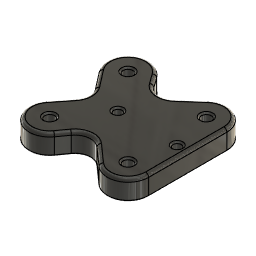
Rod_Clamp_Fixture (Autodesk Fusion 360 design; units mm, degrees)
Autodesk Fusion 360 part; units mm, degrees
note: some values were not read from the file. Set by a fixed rule: which sketch regions a step uses.
sketch "Sketch1" plane through (0, 0, 0) normal (0, 0, 1) x (1, 0, 0)
  circle A0 centre (0, 0) radius 3.125
  circle A1 centre (0, 50) radius 3.125
  circle A2 centre (0, 0) radius 13.125
  circle A3 centre (0, 50) radius 13.125
  line L0 (0, 50) -> (0, 0) construction
  line L1 (37.5, 50.1021) -> (37.5, 0.1021) construction
  line L2 (0, 25) -> (18.55, 25) construction
  circle A4 centre (18.55, 25) radius 2.6
  circle A5 centre (18.55, 25) radius 12.6 construction
  line L3 (-10.2863, 8.1521) -> (-1.9703, 18.6453)
  line L4 (-1.8904, 30.9655) -> (-10.3911, 41.9818)
  arc A6 (-1.9703, 18.6453) -> (-1.8904, 30.9655) centre (-9.8074, 24.8564) ccw
  line L5 (75, 25) -> (56.45, 25) construction
  circle A7 centre (56.45, 25) radius 2.6
  circle A8 centre (56.45, 25) radius 12.6 construction
  line L6 (10.6707, 57.6421) -> (15.1766, 51.3504)
  line L7 (50, 25) -> (50, 37.5) construction
  line L8 (0, 0) -> (37.5, 0) construction
  line L9 (18.55, 25) -> (56.45, 25) construction
  line L10 (37.5, 25) -> (37.5, 37.5) construction
  circle A9 centre (50.0503, 50) radius 13.125
  circle A10 centre (50.0503, 50) radius 3.125
  circle A11 centre (50.0503, 0) radius 13.125
  circle A12 centre (50.0503, 0) radius 3.125
  line L11 (29.9485, 49.6973) -> (41.3329, 59.8118)
  line L12 (21.6444, 42.3194) -> (21.6444, 45)
  line L13 (0, 50) -> (50.0503, 50) construction
  arc A13 (15.1766, 51.3504) -> (29.9485, 49.6973) centre (23.3067, 57.173) ccw
  line L14 (63.1753, 50) -> (63.1753, 0)
  line L15 (56.45, 25) -> (61.45, 25) construction
  arc A14 (29.9485, 0.3027) -> (15.1766, -1.3504) centre (23.3067, -7.173) ccw
  line L16 (10.6707, -7.6421) -> (15.1766, -1.3504)
  line L17 (29.9485, 0.3027) -> (41.3329, -9.8118)
  point P0 (5.95, 25)
  dimension "d156" = 6.25
  dimension "d159" = 25
  dimension "d160" = 25
  dimension "d161" = 10
  dimension "d162" = 10
  dimension "d163" = 50
  dimension "d165" = 50
  dimension "d166" = 18.55
  dimension "d167" = 5.2
  dimension "d168" = 10
  dimension "d169" = 10
  dimension "d178" = 37.5
  dimension "d5" = 25
  dimension "d6" = 25
  dimension "d7" = 10
  dimension "d8" = 10
  dimension "d9" = 6.25
  dimension "d10" = 50
  dimension "d11" = 10
  dimension "d12" = 5
  constraint coincident A0.centre A2.centre
  constraint coincident A1.centre A3.centre
  constraint midpoint L0 L2.start
  constraint vertical L1
  constraint perpendicular L0 L2
  constraint coincident L2.end A4.centre
  constraint coincident A2 L3.start
  constraint tangent A2 L3
  constraint coincident A5 P0
  constraint coincident A3 L4.end
  constraint tangent A3 L4
  constraint tangent L4 A6
  constraint tangent L3 A6
  constraint symmetric L1 L2.end L5.end
  constraint symmetric L1 A4 A7
  constraint symmetric L1 A5 A8
  constraint tangent A5 L6
  constraint coincident A3 L6.start
  constraint tangent A3 L6
  constraint perpendicular L1 L8
  constraint coincident L1 L8.end
  constraint midpoint L9 L10.start
  constraint coincident A9 L11.end
  constraint tangent A9 L11
  constraint vertical L12
  constraint coincident A9.centre A10.centre
  constraint perpendicular L0 L13
  constraint coincident L6 L12.start
  constraint coincident L12.start L11
  constraint tangent L6 A13
  constraint tangent L11 A13
  constraint coincident A9 L14.start
  constraint coincident A11 L14.end
  constraint tangent A11 L14
  constraint coincident L5.end A7.centre
  constraint perpendicular L14 L15
  constraint symmetric L2 L6.start L16.start
  constraint symmetric L2 L11.end L17.end
  constraint symmetric L2 L6.end A14.end
  constraint symmetric L2 L11.start A14.start
  constraint symmetric L2 A13 A14
  constraint tangent A9 L14
  measures "d156" diameter of A0
  measures "d163" distance of A1.centre A0.centre
  measures "d165" distance of L2.start L7.start
  measures "d166" distance of L2.start L2.end
  measures "d167" diameter of A4
  measures "d169" radius of A6
  measures "d178" distance of A0.centre L8.end
  measures "d9" diameter of A12
  measures "d10" distance of A9.centre A11.centre
  measures "d11" radius of A13
  measures "d12" distance of L5.end L15.end
extrude "Extrude1" add sketch "Sketch1" along normal blind 12.5
chamfer "Chamfer1" distance 1 angle 45 6 edges at (-2.9135, 51.13, 12.5) (47.1368, 51.13, 12.5) (54.0259, 25.9402, 12.5) (16.1259, 25.9402, 12.5) (47.1368, 1.13, 12.5) (-2.9135, 1.13, 12.5)
fillet "Fillet1" radius 2 14 edges at (12.9237, 54.4962, 12.5) (-7.8314, 60.5326, 12.5) (-6.1408, 36.4737, 12.5) (0.1923, 24.7916, 12.5) (-6.1283, 13.3987, 12.5) (-7.8994, -10.4816, 12.5) (12.9237, -4.4962, 12.5) (22.1945, 2.765, 12.5) (35.6407, -4.7546, 12.5) (55.4285, -11.9725, 12.5) (63.1753, 25, 12.5) (22.1945, 47.235, 12.5) (35.6407, 54.7546, 12.5) (55.4285, 61.9725, 12.5)
sketch "Sketch2" plane through (0, 0, 0) normal (0, 0, -1) x (1, 0, 0)
  circle A0 centre (0, 0) radius 3.125
  line L0 (22.6, -22.6617) -> (18.55, -20.3235)
  line L1 (18.55, -20.3235) -> (14.5, -22.6617)
  line L2 (14.5, -22.6617) -> (14.5, -27.3383)
  line L3 (14.5, -27.3383) -> (18.55, -29.6765)
  line L4 (18.55, -29.6765) -> (22.6, -27.3383)
  line L5 (22.6, -27.3383) -> (22.6, -22.6617)
  circle A1 centre (50.0503, 0) radius 3.125
  circle A2 centre (0, -50) radius 3.125
  circle A3 centre (56.45, -25) radius 2.6
  circle A4 centre (50.0503, -50) radius 3.125
  circle A5 centre (18.55, -25) radius 2.6
  arc A6 (10.6707, 7.6421) -> (-10.2863, -8.1521) centre (0, 0) ccw
  line L6 (-10.2863, -8.1521) -> (-1.9703, -18.6453)
  arc A7 (-1.8904, -30.9655) -> (-1.9703, -18.6453) centre (-9.8074, -24.8564) ccw
  line L7 (-1.8904, -30.9655) -> (-10.3911, -41.9818)
  arc A8 (-10.3911, -41.9818) -> (10.6707, -57.6421) centre (0, -50) ccw
  line L8 (10.6707, -57.6421) -> (15.1766, -51.3504)
  arc A9 (29.9485, -49.6973) -> (15.1766, -51.3504) centre (23.3067, -57.173) ccw
  line L9 (29.9485, -49.6973) -> (41.3329, -59.8118)
  arc A10 (41.3329, -59.8118) -> (63.1753, -50) centre (50.0503, -50) ccw
  line L10 (63.1753, -50) -> (63.1753, 0)
  arc A11 (63.1753, 0) -> (41.3329, 9.8118) centre (50.0503, 0) ccw
  line L11 (41.3329, 9.8118) -> (29.9485, -0.3027)
  arc A12 (15.1766, 1.3504) -> (29.9485, -0.3027) centre (23.3067, 7.173) ccw
  line L12 (15.1766, 1.3504) -> (10.6707, 7.6421)
  point P0 (18.55, -25)
  dimension "d194" = 4.05
  constraint parallel L5 L10
  constraint coincident P0 A5.centre
  measures "d194" distance of P0 L5
extrude "Extrude2" cut sketch "Sketch2" against normal blind 4.5 contours L0 L1 L2 L3 L4 L5
ref_plane "WorkPlane2" through (37.5, 0, 0) normal (1, 0, 0) x (0, 1, 0)
mirror "Mirror5" about plane through (37.5, 0, 0) normal (1, 0, 0) of "Extrude2"
chamfer "Chamfer2" distance 0.5 angle 45 14 edges at (55.4285, -11.9725, 0) (63.1753, 25, 0) (55.4285, 61.9725, 0) (35.6407, 54.7546, 0) (22.1945, 47.235, 0) (12.9237, 54.4962, 0) (-7.8314, 60.5326, 0) (-6.1408, 36.4737, 0) (0.1923, 24.7916, 0) (-6.1283, 13.3987, 0) (-7.8994, -10.4816, 0) (12.9237, -4.4962, 0) (22.1945, 2.765, 0) (35.6407, -4.7546, 0)
equation "d156 = Print6mmOD"
equation "d178 = ( 75 / 2 ) * 1 mm"
equation "d198 = ( 75 / 2 ) * 1 mm"
equation "d9 = Print6mmOD"
equation "Print6mmOD = 6.25 mm" comment "3D Printing"
